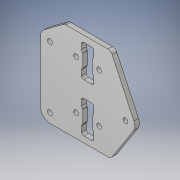
# Autodesk Inventor part: 上昇機構_外側板
Saved by Autodesk Inventor 2019.4 (Build 234330000, 330)
## iProperties
Created: 2021-12-04
Part Number: 上昇機構_外側板
Material: アルミニウム 6061
Document SubType Name: Modeling
Designer: 堀川皓史
Density: 2.7 g/cm^3
Appearance: アルミニウム - フラット
Author: 堀川皓史
Autodesk Inventor part; units mm, degrees
ref_plane "YZ Plane" through (0, 0, 0) normal (1, 0, 0) x (0, 1, 0)
ref_plane "XZ Plane" through (0, 0, 0) normal (0, 1, 0) x (-1, 0, 0)
ref_plane "XY Plane" through (0, 0, 0) normal (0, 0, 1) x (1, 0, 0)
sketch "スケッチ1" plane through (0, 0, 0) normal (0, 0, 1) x (1, 0, 0)
  line L0 (-15, 61.424) -> (15, 61.424) construction
  line L1 (15, 61.424) -> (15, -32.317) construction
  line L2 (15, -32.317) -> (-15, -32.317) construction
  line L3 (-15, -32.317) -> (-15, 61.424) construction
  circle A0 centre (-24.5, 20) radius 9.5 construction
  circle A1 centre (24.5, 0) radius 9.5 construction
  circle A2 centre (-24.5, -20) radius 9.5 construction
  line L4 (-24.5, 20) -> (24.5, 0) construction
  line L5 (24.5, 0) -> (-24.5, -20) construction
  line L6 (-24.5, -20) -> (-24.5, 20) construction
  circle A3 centre (-24.5, 20) radius 1.6
  circle A4 centre (24.5, 0) radius 1.6
  circle A5 centre (-24.5, -20) radius 1.6
  line L7 (-3, 29.5) -> (3, 29.5) construction
  line L8 (3, 29.5) -> (3, 10.5) construction
  line L9 (3, 10.5) -> (-3, 10.5) construction
  line L10 (-3, 10.5) -> (-3, 29.5) construction
  circle A6 centre (-7.5, 20) radius 1.6
  circle A7 centre (7.5, 20) radius 1.6
  line L11 (-2.5, 9.5) -> (2.5, 9.5)
  line L12 (4, 11) -> (4, 14.3297)
  line L13 (2.5, 30.5) -> (-2.5, 30.5)
  line L14 (-3.1, 24) -> (-3.1, 16)
  line L15 (3.1, 24) -> (3.1, 16)
  line L16 (-4, 14.3297) -> (-4, 11)
  line L17 (4, 25.6703) -> (4, 29)
  arc A8 (-2.5, 30.5) -> (-4, 29) centre (-2.5, 29) ccw
  arc A9 (4, 29) -> (2.5, 30.5) centre (2.5, 29) ccw
  arc A10 (-4, 11) -> (-2.5, 9.5) centre (-2.5, 11) ccw
  arc A11 (2.5, 9.5) -> (4, 11) centre (2.5, 11) ccw
  line L18 (-4, 29) -> (-4, 25.6703)
  arc A12 (-4, 25.6703) -> (-3.325, 24.4176) centre (-2.5, 25.6703) ccw
  arc A13 (-3.1, 24) -> (-3.325, 24.4176) centre (-3.6, 24) ccw
  arc A14 (3.325, 24.4176) -> (4, 25.6703) centre (2.5, 25.6703) ccw
  arc A15 (3.325, 24.4176) -> (3.1, 24) centre (3.6, 24) ccw
  arc A16 (-3.325, 15.5824) -> (-4, 14.3297) centre (-2.5, 14.3297) ccw
  arc A17 (-3.325, 15.5824) -> (-3.1, 16) centre (-3.6, 16) ccw
  arc A18 (3.1, 16) -> (3.325, 15.5824) centre (3.6, 16) ccw
  arc A19 (4, 14.3297) -> (3.325, 15.5824) centre (2.5, 14.3297) ccw
  circle A20 centre (-7.5, -11.5) radius 1.6
  line L19 (-3.1, -7.5) -> (-3.1, -15.5)
  line L20 (3.1, -7.5) -> (3.1, -15.5)
  circle A21 centre (7.5, -11.5) radius 1.6
  line L21 (3, -21) -> (-3, -21) construction
  arc A22 (2.5, -22) -> (4, -20.5) centre (2.5, -20.5) ccw
  arc A23 (3.1, -15.5) -> (3.325, -15.9176) centre (3.6, -15.5) ccw
  line L22 (4, -20.5) -> (4, -17.1703)
  arc A24 (4, -17.1703) -> (3.325, -15.9176) centre (2.5, -17.1703) ccw
  arc A25 (-3.325, -15.9176) -> (-3.1, -15.5) centre (-3.6, -15.5) ccw
  line L23 (-3, -2) -> (3, -2) construction
  line L24 (3, -2) -> (3, -21) construction
  arc A26 (-3.325, -15.9176) -> (-4, -17.1703) centre (-2.5, -17.1703) ccw
  line L25 (-4, -17.1703) -> (-4, -20.5)
  arc A27 (-4, -20.5) -> (-2.5, -22) centre (-2.5, -20.5) ccw
  line L26 (-3, -21) -> (-3, -2) construction
  line L27 (2.5, -1) -> (-2.5, -1)
  line L28 (4, -5.8297) -> (4, -2.5)
  arc A28 (-2.5, -1) -> (-4, -2.5) centre (-2.5, -2.5) ccw
  arc A29 (3.325, -7.0824) -> (3.1, -7.5) centre (3.6, -7.5) ccw
  arc A30 (-3.1, -7.5) -> (-3.325, -7.0824) centre (-3.6, -7.5) ccw
  arc A31 (-4, -5.8297) -> (-3.325, -7.0824) centre (-2.5, -5.8297) ccw
  arc A32 (3.325, -7.0824) -> (4, -5.8297) centre (2.5, -5.8297) ccw
  line L29 (-4, -2.5) -> (-4, -5.8297)
  arc A33 (4, -2.5) -> (2.5, -1) centre (2.5, -2.5) ccw
  line L30 (-2.5, -22) -> (2.5, -22)
  line L31 (-15, 34.5) -> (15, 34.5)
  line L32 (-24.5, -26) -> (15, -26)
  arc A34 (-28.0705, 24.822) -> (-30.5, 20) centre (-24.5, 20) ccw
  arc A35 (-30.5, -20) -> (-24.5, -26) centre (-24.5, -20) ccw
  arc A36 (29.5553, -3.2317) -> (29.9357, 2.5403) centre (24.5, 0) ccw
  line L33 (-15, 34.5) -> (-28.0705, 24.822)
  line L34 (-30.5, 20) -> (-30.5, -20)
  line L35 (15, -26) -> (29.5553, -3.2317)
  line L36 (15, 34.5) -> (29.9357, 2.5403)
  point P0 (0, 0)
  point P1 (0, 20)
  point P2 (0, -11.5)
  dimension "d0" = 30
  dimension "d1" = 15
  dimension "d2" = 19
  dimension "d3" = 19
  dimension "d4" = 19
  dimension "d5" = 40
  dimension "d7" = 3.2
  dimension "d8" = 3.2
  dimension "d9" = 3.2
  dimension "d10" = 6
  dimension "d11" = 19
  dimension "d12" = 3
  dimension "d13" = 9.5
  dimension "d14" = 3.2
  dimension "d15" = 3.2
  dimension "d16" = 15
  dimension "d17" = 7.5
  dimension "d18" = 1
  dimension "d19" = 8
  dimension "d20" = 4
  dimension "d21" = 0.1
  dimension "d22" = 0.1
  dimension "d23" = 1
  dimension "d24" = 1
  dimension "d25" = 1
  dimension "d26" = 1.5
  dimension "d27" = 1
  dimension "d28" = 1.5
  dimension "d29" = 0.5
  dimension "d30" = 1
  dimension "d31" = 1.5
  dimension "d32" = 0.5
  dimension "d33" = 1.5
  dimension "d34" = 0.5
  dimension "d35" = 0.5
  dimension "d36" = 1.5
  dimension "d37" = 6
  dimension "d38" = 19
  dimension "d39" = 3
  dimension "d40" = 9.5
  dimension "d41" = 3.2
  dimension "d42" = 3.2
  dimension "d43" = 15
  dimension "d44" = 7.5
  dimension "d45" = 1
  dimension "d46" = 8
  dimension "d47" = 4
  dimension "d48" = 0.1
  dimension "d49" = 0.1
  dimension "d50" = 1
  dimension "d51" = 1
  dimension "d52" = 1
  dimension "d53" = 1.5
  dimension "d54" = 1
  dimension "d55" = 1.5
  dimension "d56" = 0.5
  dimension "d57" = 1
  dimension "d58" = 1.5
  dimension "d59" = 0.5
  dimension "d60" = 1.5
  dimension "d61" = 0.5
  dimension "d62" = 0.5
  dimension "d63" = 1.5
  dimension "d64" = 4
  constraints: 74 end point, 54 point on circle, 46 tangent, 37 centre point, 14 horizontal alignment, 12 parallel, 7 perpendicular, 7 vertical, 6 coincident, 6 equal radius, 5 horizontal, 3 vertical alignment, 2 point on line, 1 equal length
  measures "d0" distance between parallel lines of L1 L3
  measures "d1" distance from line of point (0, 0) L3
  measures "d2" diameter of A0
  measures "d3" diameter of A1
  measures "d4" diameter of A2
  measures "d5" distance of L5.end L4.start
  measures "d7" diameter of A3
  measures "d8" diameter of A4
  measures "d9" diameter of A5
  measures "d10" distance of L7.start L7.end
  measures "d11" distance of L7.end L9.start
  measures "d12" distance from line of point (0, 20) L10
  measures "d13" distance from line of point (0, 20) L7
  measures "d14" diameter of A6
  measures "d15" diameter of A7
  measures "d16" distance of A7.centre A6.centre
  measures "d17" distance of point (0, 20) A6.centre
  measures "d18" distance between parallel lines of L9 L11
  measures "d19" distance of L14.start L14.end
  measures "d20" vertical distance of point (0, 20) L14.end
  measures "d21" distance between parallel lines of L14 L10
  measures "d22" distance between parallel lines of L8 L15
  measures "d23" distance between parallel lines of L10 L16
  measures "d24" distance between parallel lines of L8 L12
  measures "d25" distance between parallel lines of L7 L13
  measures "d26" radius of A8
  measures "d27" distance between parallel lines of L10 L18
  measures "d28" radius of A12
  measures "d29" radius of A13
  measures "d30" distance between parallel lines of L8 L17
  measures "d31" radius of A14
  measures "d32" radius of A15
  measures "d33" radius of A16
  measures "d34" radius of A17
  measures "d35" radius of A18
  measures "d36" radius of A19
  measures "d37" distance of L26.end L24.start
  measures "d38" distance of L24.start L24.end
  measures "d39" distance from line of point (0, -11.5) L26
  measures "d40" distance from line of point (0, -11.5) L23
  measures "d41" diameter of A20
  measures "d42" diameter of A21
  measures "d43" distance of A21.centre A20.centre
  measures "d44" distance of point (0, -11.5) A20.centre
  measures "d45" distance between parallel lines of L21 L30
  measures "d46" distance of L19.start L19.end
  measures "d47" vertical distance of point (0, -11.5) L19.end
  measures "d48" distance between parallel lines of L19 L26
  measures "d49" distance between parallel lines of L24 L20
  measures "d50" distance between parallel lines of L26 L25
  measures "d51" distance between parallel lines of L24 L22
  measures "d52" distance between parallel lines of L23 L27
  measures "d53" radius of A28
  measures "d54" distance between parallel lines of L26 L29
  measures "d55" radius of A31
  measures "d56" radius of A30
  measures "d57" distance between parallel lines of L24 L28
  measures "d58" radius of A32
  measures "d59" radius of A29
  measures "d60" radius of A26
  measures "d61" radius of A25
  measures "d62" radius of A23
  measures "d63" radius of A24
  measures "d64" distance between parallel lines of L13 L31
extrude "押し出し1" add sketch "スケッチ1" along normal blind 3
fillet "フィレット1" radius 3 3 edges at (-15, 34.5, 1.5) (15, 34.5, 1.5) (15, -26, 1.5)
equation "\"d1\" = 0.5 * d0"
equation "\"d13\" = 0.5 * d11"
equation "\"d17\" = 0.5 * d16"
equation "\"d40\" = 0.5 * d38"
equation "\"d44\" = 0.5 * d43"
